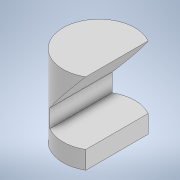
# Autodesk Inventor part: Деталь3
Saved by Autodesk Inventor 2021.2 (Build 252289000, 289)
## iProperties
Created: 2023-10-05
Part Number: Деталь3
Material: Типовые
Document SubType Name: Modeling
Designer: User
Density: 1 g/cm^3
Appearance: По умолчанию
Author: User
Autodesk Inventor part; units mm, degrees
ref_plane "YZ Plane" through (0, 0, 0) normal (1, 0, 0) x (0, 1, 0)
ref_plane "XZ Plane" through (0, 0, 0) normal (0, 1, 0) x (-1, 0, 0)
ref_plane "XY Plane" through (0, 0, 0) normal (0, 0, 1) x (1, 0, 0)
sketch "Эскиз1" plane through (0, 0, 0) normal (0, 1, 0) x (-1, 0, 0)
  circle A0 centre (0, 0) radius 40
  dimension "d0" = 80
  constraints: 1 centre point, 1 coincident
  measures "d0" diameter of A0
extrude "Выдавливание1" add sketch "Эскиз1" along normal blind 90
sketch "Эскиз2" plane through (0, 0, 0) normal (0, 0, 1) x (1, 0, 0)
  line L0 (-40, 90) -> (-40, 0)
  line L1 (-40, 0) -> (-40, 90) projected
  line L2 (-40, 0) -> (20, 0)
  line L3 (20, 0) -> (20, 20)
  line L4 (20, 20) -> (-20, 20)
  line L5 (-20, 20) -> (-20, 40)
  line L6 (-20, 40) -> (20, 90)
  line L7 (20, 90) -> (-40, 90)
  point P0 (0, 0)
  dimension "d3" = 60
  dimension "d4" = 20
  dimension "d5" = 40
  dimension "d6" = 20
  constraints: 14 end point, 3 perpendicular, 2 point on line
  measures "d3" distance of L1.start L2.end
  measures "d4" distance of L2.end L3.end
  measures "d5" distance of L3.end L4.end
  measures "d6" distance of L4.end L5.end
extrude "Выдавливание2" cut sketch "Эскиз2" against normal mid plane 90 keep common part
